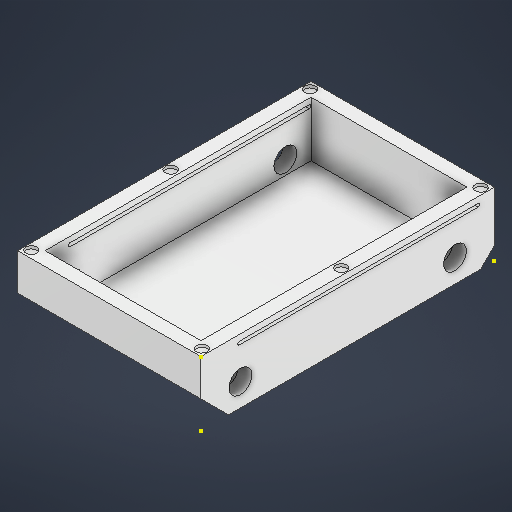
# Autodesk Inventor part: Body
Saved by Autodesk Inventor 2027 (Build 310192060, 192F)
## iProperties
Created: 2026-06-05
Part Number: Body
Material: ABS Plastic
Document SubType Name: Modeling
Designer: CatKartikSUPREMEPC
Mass: 1509.41 g
Surface Area: 2492.64 cm^2
Volume: 1423.97 cm^3
Density: 1.06 g/cm^3
Appearance: Smooth - White
Author: CatKartikSUPREMEPC
Autodesk Inventor part; units mm, degrees
ref_plane "YZ Plane" through (0, 0, 0) normal (1, 0, 0) x (0, 1, 0)
ref_plane "XZ Plane" through (0, 0, 0) normal (0, 1, 0) x (-1, 0, 0)
ref_plane "XY Plane" through (0, 0, 0) normal (0, 0, 1) x (1, 0, 0)
sketch "Sketch1" plane through (0, 0, 0) normal (0, 1, 0) x (-1, 0, 0)
  line L0 (0, 0) -> (200, 0)
  line L1 (200, 0) -> (200, -320)
  line L2 (200, -320) -> (0, -320)
  line L3 (0, -320) -> (0, 0)
  dimension "d0" = 200
  dimension "d1" = 320
  constraints: 8 end point, 2 parallel, 1 horizontal, 1 perpendicular
  measures "d0" distance of L1.end L2.end
  measures "d1" distance of L2.end L0.start
extrude "Extrusion1" add sketch "Sketch1" along normal blind 70
chamfer "Chamfer1" distance 30 angle 45 1 edges at (-100, 0, 0)
shell "Shell1" thickness 15 removed faces 1 at (-66.6667, 70, -106.6667)
sketch "Sketch5" plane through (0, 70, 0) normal (0, 1, 0) x (1, 0, 0)
  circle A0 centre (-192.9908, 160) radius 6
  line L0 (-200, 0) -> (0, 0) projected
  circle A1 centre (-192.9908, 8) radius 6
  circle A2 centre (-192.9908, 312) radius 6
  line L1 (-100, -14.4089) -> (-100, 373.6947) construction
  circle A3 centre (-7.0092, 160) radius 6
  circle A4 centre (-7.0092, 8) radius 6
  circle A5 centre (-7.0092, 312) radius 6
  dimension "d40" = 12
  dimension "d41" = 160
  dimension "d42" = 12
  dimension "d43" = 152
  dimension "d44" = 12
  dimension "d45" = 152
  constraints: 6 centre point, 3 symmetric about line, 2 end point, 1 vertical, 3 other
  measures "d40" diameter of A0
  measures "d41" distance from line of A0.centre L0
  measures "d42" diameter of A1
  measures "d43" distance of A0.centre A1.centre
  measures "d44" diameter of A2
  measures "d45" distance of A2.centre A0.centre
extrude "Extrusion5" cut sketch "Sketch5" against normal blind 3
chamfer "Chamfer2" distance 15 angle 45 1 edges at (-100, 0, -320)
sketch "Sketch6" plane through (0, 70, 0) normal (1, 0, 0) x (0, 0, -1)
  circle A0 centre (43, -45) radius 12.5
  line L0 (0, 0) -> (320, 0) projected
  line L1 (0, -40) -> (0, 0) projected
  line L2 (320, 0) -> (0, 0) projected
  line L3 (160, 0) -> (160, -70) construction
  circle A1 centre (277, -45) radius 12.5
  point P0 (0, -70)
  dimension "d51" = 25
  dimension "d52" = 45
  dimension "d53" = 43
  constraints: 2 centre point, 2 end point, 1 midpoint, 1 symmetric about line, 1 vertical, 1 other
  measures "d51" diameter of A0
  measures "d52" distance from line of L0 A0.centre
  measures "d53" distance from line of A0.centre L1
sketch "Sketch8" plane through (-185, 15, -36.2132) normal (0, 1, 0) x (1, 0, 0)
  line L0 (170, 0) -> (170, 268.7868) projected
  line L1 (0, 0) -> (170, 0)
  line L2 (170, 0) -> (170, 268.7868)
  line L3 (170, 268.7868) -> (0, 268.7868)
  line L4 (0, 268.7868) -> (0, 0)
  point P0 (185, -36.2132)
  constraints: 8 end point, 2 parallel, 1 horizontal, 1 perpendicular
extrude "Extrusion6" cut sketch "Sketch8" against normal blind 5
sketch "Sketch9" plane through (-15, 36.2132, -15) normal (0, 0.7071068, -0.7071068) x (-1, 0, 0)
  line L0 (-0.7971, -12.8149) -> (-1.097, -36.2132)
  line L1 (185, -36.2132) -> (-15, -36.2132) projected
  line L2 (0, -33.5355) -> (170, -33.5355) projected
  line L3 (170, 23.8909) -> (170, -181.1701) projected
  line L4 (0, -33.5355) -> (170, -33.5355)
  line L5 (170, -33.5355) -> (170, -20.1439)
  line L6 (170, -20.1439) -> (0, -20.1439)
  line L7 (0, -20.1439) -> (0, -33.5355)
  point P0 (-15, -15)
  constraints: 10 end point, 2 parallel, 2 point on line, 1 horizontal, 1 perpendicular
extrude "Extrusion7" cut sketch "Sketch9" against normal blind 5
extrude "Extrusion8" cut sketch "Sketch6" against normal blind 220
sketch "Sketch10" plane through (0, 70, -320) normal (0, 0, -1) x (-1, 0, 0)
  point P0 (0, -70)
sketch "Sketch11" plane through (0, 70, -320) normal (0, 0, -1) x (-1, 0, 0)
  point P0 (0, -70)
sketch "Sketch12" plane through (0, 70, 0) normal (0, 1, 0) x (1, 0, 0)
  point P0 (0, 0)
sketch "Sketch13" plane through (0, 70, 0) normal (1, 0, 0) x (0, 0, -1)
  point P0 (0, -70)
sketch "Sketch14" plane through (0, 70, -320) normal (0, 0, -1) x (-1, 0, 0)
  point P0 (0, -70)
sketch "Sketch15" plane through (0, 70, 0) normal (1, 0, 0) x (0, 0, -1)
  point P0 (0, -70)
sketch "Sketch16" plane through (0, 70, 0) normal (1, 0, 0) x (0, 0, -1)
  line L0 (41.7462, -8.2025) -> (302.1648, -8.2025) construction
  line L1 (41.7462, -6.4667) -> (302.1648, -6.4667)
  line L2 (302.1648, -9.9384) -> (41.7462, -9.9384)
  arc A0 (41.7462, -6.4667) -> (41.7462, -9.9384) centre (41.7462, -8.2025) ccw
  arc A1 (302.1648, -9.9384) -> (302.1648, -6.4667) centre (302.1648, -8.2025) ccw
  point P0 (0, -70)
  point P1 (171.9555, -8.2025)
  constraints: 8 end point, 4 point on circle, 4 tangent, 2 centre point, 1 horizontal, 1 midpoint, 1 parallel
extrude "Extrusion10" cut sketch "Sketch16" against normal blind 20
sketch "Sketch18" plane through (-200, 70, -320) normal (-1, 0, 0) x (0, 0, 1)
  line L0 (15, -60) -> (15, 0) projected
  line L1 (277.9177, -6.1098) -> (17, -6.1098)
  line L2 (15, -8.1098) -> (15, -7.8958)
  line L3 (17, -9.8958) -> (277.9177, -9.8958)
  line L4 (279.9177, -7.8958) -> (279.9177, -8.1098)
  arc A0 (17, -6.1098) -> (15, -8.1098) centre (17, -8.1098) ccw
  arc A1 (15, -7.8958) -> (17, -9.8958) centre (17, -7.8958) ccw
  arc A2 (279.9177, -8.1098) -> (277.9177, -6.1098) centre (277.9177, -8.1098) ccw
  arc A3 (277.9177, -9.8958) -> (279.9177, -7.8958) centre (277.9177, -7.8958) ccw
  point P0 (320, -70)
  point P1 (15, -9.8958)
  point P2 (15.0029, -8.0028)
  point P3 (279.9148, -8.0028)
  dimension "d65" = 2
  constraints: 8 end point, 8 point on circle, 8 tangent, 4 centre point, 3 equal radius, 3 point on line, 2 parallel, 1 horizontal, 1 perpendicular
  measures "d65" radius of A0
extrude "Extrusion11" cut sketch "Sketch18" against normal blind 20 contours A0 L1 A2 A3 L3 A1
body "Solid1"
